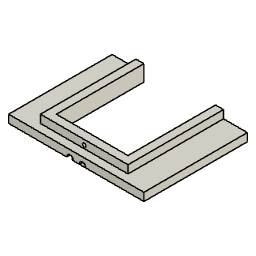
gurigri_base_plate_y_torque (Autodesk Fusion 360 design; units mm, degrees)
Autodesk Fusion 360 part; units mm, degrees
box "直方体プリミティブ1" add length 65 width 85 height 5 placed x (0, 1, 0) y (-1, 0, 0) z (0, 0, 1) at (85, 0, 0) makes body 1
sketch "スケッチ2" plane through (0, 0, 5) normal (0, 0, 1) x (-1, 0, 0)
  line L0 (-85, -65) -> (0, -65)
  line L1 (0, -65) -> (0, 0)
  line L2 (0, 0) -> (-85, 0)
  line L3 (-85, 0) -> (-85, -65)
  line L4 (0, -65) -> (-20, -65)
  line L5 (-25, -65) -> (-60, -65)
  line L6 (-65, -65) -> (-85, -65)
  line L7 (-65, -20) -> (-60, -20)
  line L8 (-60, -20) -> (-60, -65)
  line L9 (-65, -65) -> (-65, -20)
  line L10 (-25, -20) -> (-20, -20)
  line L11 (-20, -20) -> (-20, -25)
  line L12 (-20, -25) -> (-25, -25)
  line L13 (-25, -25) -> (-60, -25)
  line L14 (-65, -25) -> (-25, -25)
  line L15 (-25, -65) -> (-20, -65)
  line L16 (-60, -25) -> (-25, -25)
  line L17 (-25, -20) -> (-60, -20)
  line L18 (-25, -25) -> (-25, -65)
  line L19 (-20, -65) -> (-20, -25)
  line L20 (-25, -20) -> (-25, -25)
  constraint coincident L0.end L1.start
  constraint coincident L0 L4.end
  constraint perpendicular L1 L4
  constraint coincident L0 L5.start
  constraint coincident L0 L5.end
  constraint perpendicular L1 L5
  constraint coincident L0 L6.start
  constraint coincident L0.start L3.end
  constraint perpendicular L3 L6
  constraint perpendicular L3 L7
  constraint perpendicular L5 L8
  constraint perpendicular L7 L9
  constraint perpendicular L8 L10
  constraint perpendicular L10 L11
  constraint perpendicular L11 L12
  constraint coincident L8 L13.end
  constraint perpendicular L8 L13
  constraint coincident L9 L14.start
  constraint perpendicular L8 L14
  constraint perpendicular L8 L17
  constraint perpendicular L5 L18
  constraint perpendicular L12 L19
  constraint perpendicular L13 L20
sketch "スケッチ3" plane through (0, 0, 5) normal (0, 0, 1) x (-1, 0, 0)
  line L0 (-65, -10) -> (-20, 0)
  line L1 (-20, 0) -> (-20, -10)
  line L2 (-20, -10) -> (-65, 0)
  line L3 (-65, 0) -> (-65, -10)
  line L4 (-42.5, -5) -> (-35, -5)
  line L5 (-35, -5) -> (-35, -10)
  line L6 (-35, -10) -> (-50, -10)
  line L7 (-50, -10) -> (-50, -5)
  line L8 (-50, -5) -> (-42.5, -5)
  line L9 (-65, -10) -> (-65, -55)
  line L10 (-65, -55) -> (-60, -55)
  line L11 (-60, -55) -> (-25, -55)
  line L12 (-25, -55) -> (-20, -55)
  line L13 (-20, -55) -> (-20, -15)
  line L14 (-20, -15) -> (-25, -15)
  line L15 (-25, -15) -> (-60, -15)
  line L16 (-60, -15) -> (-65, -15)
  line L17 (-20, -15) -> (-20, -10)
  line L18 (-25, -10) -> (-60, -10)
  line L19 (-60, -10) -> (-65, -10)
  constraint vertical L1
  constraint parallel L1 L3
  constraint midpoint L2 L4.start
  constraint perpendicular L1 L4
  constraint perpendicular L4 L5
  constraint perpendicular L5 L6
  constraint perpendicular L6 L7
  constraint perpendicular L7 L8
  constraint parallel L7 L9
  constraint perpendicular L9 L10
  constraint perpendicular L9 L11
  constraint perpendicular L9 L12
  constraint perpendicular L12 L13
  constraint perpendicular L13 L14
  constraint perpendicular L13 L15
  constraint coincident L9 L16.end
  constraint perpendicular L9 L16
  constraint perpendicular L16 L17
  constraint perpendicular L17 L18
  constraint perpendicular L9 L19
box "直方体プリミティブ2" add length 40 width 35 height 5 placed x (0, -1, 0) y (1, 0, 0) z (0, 0, 1) at (25, 55, 5) separate body makes body 2
move_body "移動1" bodies 2 to x (1, 0, 0) y (0, 1, 0) z (0, 0, 1) at (0, 0, -5)
combine "結合1" operation cut target body 1 tool bodies 2
box "直方体プリミティブ3" cut length 45 width 45 height -5 placed x (0, -1, 0) y (1, 0, 0) z (0, 0, 1) at (20, 55, 5) bodies 1
box "直方体プリミティブ4" add length 5 width 15 height 15 placed x (0, -1, 0) y (1, 0, 0) z (0, 0, 1) at (35, 10, 5) bodies 1
sketch "スケッチ7" plane through (0, 5, 0) normal (0, -1, 0) x (1, 0, 0)
  line L0 (35, 20) -> (35, 5)
  line L1 (35, 5) -> (50, 5)
  line L2 (50, 5) -> (50, 20)
  line L3 (50, 20) -> (35, 20)
  line L4 (50, 20) -> (35, 5)
  line L5 (50, 5) -> (35, 20)
  circle A0 centre (42.5, 12.5) radius 4.5
  line L6 (42.5, 17) -> (38.6029, 10.25)
  line L7 (38.6029, 10.25) -> (46.3971, 10.25)
  line L8 (46.3971, 10.25) -> (42.5, 17)
  point P0 (42.5, 12.5)
  dimension "d21" = 9
  constraint coincident L2.end L3.start
  constraint coincident L0.end L1.start
  constraint coincident L1.end L2.start
  constraint coincident L0.start L3.end
  constraint midpoint L4 P0
  constraint coincident A0 L6.start
  constraint coincident P0 A0.centre
  measures "d21" diameter of A0
hole "穴1" at (38.6029, 5, 10.25) direction (0, 1, 0) diameter 2.2 depth 5 tip angle 180 bodies 1
hole "穴2" at (46.3971, 5, 10.25) direction (0, 1, 0) diameter 2.2 depth 5 tip angle 180 bodies 1
hole "穴3" at (42.5, 5, 17) direction (0, 1, 0) diameter 2.2 depth 5 tip angle 180 bodies 1
move_face "面をオフセット1" offset -10 3 faces at (61.6667, 55, 1.6667) (36.6667, 55, 1.6667) (21.6667, 55, 1.6667) on bodies 1
split "分割1" by plane through (85, 0, 5) normal (0, 0, 1) bodies 1 makes body 3 at (38.2354, 10, 16.0188)
sketch "スケッチ12" plane through (0, 5, 0) normal (0, -1, 0) x (1, 0, 0)
  line L0 (50, 5) -> (35, 5)
  line L1 (35, 5) -> (42.3217, 5)
  line L2 (50, 5) -> (42.5, 5)
  line L3 (35, 5) -> (42.5, 5)
  constraint horizontal L0
  constraint coincident L0 L1.end
  constraint midpoint L0 L2.end
  constraint parallel L2 L3
sketch "スケッチ13" plane through (0, 5, 0) normal (0, -1, 0) x (1, 0, 0)
  line L0 (50, 5) -> (35, 5)
  line L1 (35, 5) -> (42.5, 5)
  constraint horizontal L0
  constraint midpoint L0 L1.end
  constraint parallel L0 L1
sketch "スケッチ14" plane through (0, 5, 0) normal (0, -1, 0) x (1, 0, 0)
  line L0 (50, 5) -> (42.5, 5)
  line L1 (42.5, 5) -> (35, 5)
  line L2 (35, 5) -> (42.5, 5)
  constraint horizontal L0
  constraint parallel L0 L1
move_body "移動2" bodies 1 to x (1, 0, 0) y (0, 1, 0) z (0, 0, 1) at (0, 0, 10)
copy_body "ボディのコピーと貼り付け1" bodies 3 makes body 4
delete_face "面を削除1" 1 faces at (46.5066, 6.6667, 9.1555) on bodies 4
delete_face "面を削除2" 1 faces at (38.7124, 6.6667, 9.1555) on bodies 4
delete_face "面を削除3" 1 faces at (42.6095, 6.6667, 15.9055) on bodies 4
copy_body "ボディのコピーと貼り付け2" bodies 1 makes body 5
combine "結合2" operation cut target body 5 tool bodies 4
sketch "スケッチ15" plane through (0, 5, 0) normal (0, -1, 0) x (1, 0, 0)
cylinder "円柱プリミティブ1" add diameter 4 height 5 placed x (1, 0, 0) y (0, 0, 1) z (0, -1, 0) at (42.5, 5, 17) separate body makes body 6
sketch "スケッチ17" plane through (0, 5, 0) normal (0, -1, 0) x (1, 0, 0)
cylinder "円柱プリミティブ2" add diameter 4 height 10 placed x (1, 0, 0) y (0, 0, -1) z (0, 1, 0) at (46.4, 0, 10.25) separate body makes body 7
sketch "スケッチ19" plane through (0, 65, 0) normal (0, 1, 0) x (-1, 0, 0)
  line L0 (-20, 15) -> (-20, 10)
  line L1 (-20, 10) -> (0, 10)
  line L2 (0, 10) -> (0, 15)
  line L3 (0, 15) -> (-20, 15)
cylinder "円柱プリミティブ3" add diameter 4 height 10 placed x (1, 0, 0) y (0, 0, -1) z (0, 1, 0) at (38.6034, 0, 10.2499) separate body makes body 8
move_body "移動3" bodies 8 to x (1, 0, 0) y (0, 1, 0) z (0, 0, 1) at (0, -5, 0)
move_body "移動4" bodies 7 to x (1, 0, 0) y (0, 1, 0) z (0, 0, 1) at (0, -5, 0)
move_face "面をオフセット2" offset -5 1 faces at (39.0336, -5, 10.1851) on bodies 8
move_face "面をオフセット3" offset -5 1 faces at (46.8301, -5, 10.1852) on bodies 7
box "直方体プリミティブ9" add length 60 width 5 height 5 placed x (0, 1, 0) y (-1, 0, 0) z (0, 0, 1) at (20, 5, 15) separate body makes body 9
box "直方体プリミティブ10" add length 60 width 5 height 5 placed x (0, 1, 0) y (-1, 0, 0) z (0, 0, 1) at (70, 5, 15) separate body makes body 10
box "直方体プリミティブ11" add length 5 width 15 height 5 placed x (0, -1, 0) y (1, 0, 0) z (0, 0, 1) at (20, 10, 15) separate body makes body 11
box "直方体プリミティブ12" add length 5 width 15 height 5 placed x (0, 1, 0) y (-1, 0, 0) z (0, 0, 1) at (65, 5, 15) separate body makes body 12
combine "結合3" operation add target body 9 tool bodies 5 3 10 11 12
combine "結合4" operation cut target body 9 tool bodies 8 7 6
delete_body "RemoveBody1" bodies 1
